rtxsupport (Autodesk Fusion 360 design; units mm, degrees)
Autodesk Fusion 360 part; units mm, degrees
sketch "Sketch1" plane through (0, 0, 0) normal (0, 1, 0) x (1, 0, 0)
  line L0 (-70, 0) -> (50, 0)
  line L1 (-70, 0) -> (-70, 20)
  line L2 (-70, 20) -> (-80, 20)
  line L3 (-80, 20) -> (-80, -20)
  line L4 (-80, -20) -> (50.3493, -2.6201)
  line L5 (50, 0) -> (50.3493, -2.6201)
  line L6 (-70.3109, -13.2) -> (-62.1109, -13.2)
  line L7 (-62.1109, -13.2) -> (-62.1109, -5)
  line L8 (-62.1109, -5) -> (-70.3109, -5)
  line L9 (-70.3109, -5) -> (-70.3109, -13.2)
  line L10 (-9.6566, -8.2) -> (-4.4566, -8.2)
  line L11 (-4.4566, -8.2) -> (-4.4566, -3)
  line L12 (-4.4566, -3) -> (-9.6566, -3)
  line L13 (-9.6566, -3) -> (-9.6566, -8.2)
  dimension "d1" = 20
  dimension "d2" = 10
  dimension "d3" = 40
  dimension "d4" = 8.2
  dimension "d5" = 8.2
  dimension "d6" = 5
  dimension "d7" = 5.2
  dimension "d8" = 5.2
  dimension "d9" = 3
  constraint horizontal L0
  constraint perpendicular L0 L1
  constraint perpendicular L1 L2
  constraint perpendicular L2 L3
  constraint perpendicular L4 L5
  constraint horizontal L6
  constraint vertical L7
  constraint horizontal L8
  constraint vertical L9
  constraint horizontal L10
  constraint vertical L11
  constraint horizontal L12
  constraint vertical L13
  measures "d1" distance of L0.start L1.end
  measures "d2" distance of L1.end L2.end
  measures "d3" distance of L2.end L3.end
  measures "d4" distance of L6.start L6.end
  measures "d5" distance of L6.start L8.end
  measures "d6" distance of L0 L8
  measures "d7" distance of L10.start L10.end
  measures "d8" distance of L10.start L12.end
  measures "d9" distance of L0 L12
extrude "Extrude1" add sketch "Sketch1" along normal blind 8
fillet "Fillet1" radius 2 1 edges at (-70, 4, 0)
fillet "Fillet2" radius 6 1 edges at (-80, 4, -20)
fillet "Fillet3" radius 2.5 1 edges at (-70, 4, -20)
fillet "Fillet4" radius 2.5 1 edges at (-80, 4, 20)
fillet "Fillet5" radius 1.2 2 edges at (50.3493, 4, 2.6201) (50, 4, 0)
